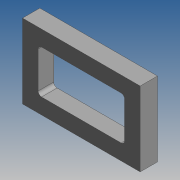
# Autodesk Inventor part: P031_MonoVitreBas
Saved by Autodesk Inventor 2021.3 (Build 253353000, 353)
## iProperties
Created: 2021-11-12
Part Number: P031_MonoVitreBas
Material: Générique
Document SubType Name: Modeling
Designer: gabri
Density: 1 g/cm^3
Appearance: Par défaut
Author: gabri
Autodesk Inventor part; units mm, degrees
ref_plane "YZ Plane" through (0, 0, 0) normal (1, 0, 0) x (0, 1, 0)
ref_plane "XZ Plane" through (0, 0, 0) normal (0, 1, 0) x (-1, 0, 0)
ref_plane "XY Plane" through (0, 0, 0) normal (0, 0, 1) x (1, 0, 0)
sketch "Sketch2" plane through (0, 0, 0) normal (0, 1, 0) x (-1, 0, 0)
  line L0 (-25, -12.5) -> (25, -12.5)
  line L1 (25, -12.5) -> (25, 12.5)
  line L2 (25, 12.5) -> (-25, 12.5)
  line L3 (-25, 12.5) -> (-25, -12.5)
  line L4 (-25, -12.5) -> (25, 12.5) construction
  line L5 (25, -12.5) -> (-25, 12.5) construction
  line L6 (-34, -21.5) -> (34, -21.5)
  line L7 (34, -21.5) -> (34, 21.5)
  line L8 (34, 21.5) -> (-34, 21.5)
  line L9 (-34, 21.5) -> (-34, -21.5)
  line L10 (-34, -21.5) -> (34, 21.5) construction
  line L11 (34, -21.5) -> (-34, 21.5) construction
  point P0 (0, 0)
  dimension "d0" = 50
  dimension "d1" = 25
  dimension "d4" = 9
  dimension "d5" = 9
  dimension "d53" = 68
  dimension "d54" = 43
  constraints: 24 end point, 4 midpoint, 4 parallel, 2 horizontal, 2 perpendicular
  measures "d0" distance of L1.end L2.end
  measures "d1" distance of L0.end L1.end
  measures "d4" distance between parallel lines of L8 L2
  measures "d5" distance between parallel lines of L1 L7
  measures "d53" distance of L6.start L6.end
  measures "d54" distance of L8.end L6.start
extrude "Extrusion1" add sketch "Sketch2" along normal blind 10
sketch "Sketch4" plane through (0, 10, 0) normal (0, 1, 0) x (1, 0, 0)
  line L0 (-34, 21.5) -> (-34, -21.5) construction
  line L1 (-34, -21.5) -> (34, -21.5) construction
  line L2 (34, -21.5) -> (34, 21.5) construction
  line L3 (34, 21.5) -> (-34, 21.5) construction
  line L4 (25, 12.5) -> (25, -12.5) construction
  line L5 (25, -12.5) -> (-25, -12.5) construction
  line L6 (-25, -12.5) -> (-25, 12.5) construction
  line L7 (-25, 12.5) -> (25, 12.5) construction
  line L8 (-25, 12.5) -> (25, 12.5)
  line L9 (25, 12.5) -> (25, -12.5)
  line L10 (25, -12.5) -> (-25, -12.5)
  line L11 (-25, -12.5) -> (-25, 12.5)
  line L12 (-25, 12.5) -> (25, -12.5) construction
  line L13 (25, 12.5) -> (-25, -12.5) construction
  line L14 (-29, 16.5) -> (29, 16.5)
  line L15 (29, 16.5) -> (29, -16.5)
  line L16 (29, -16.5) -> (-29, -16.5)
  line L17 (-29, -16.5) -> (-29, 16.5)
  line L18 (-29, 16.5) -> (29, -16.5) construction
  line L19 (29, 16.5) -> (-29, -16.5) construction
  point P0 (0, 0)
  dimension "d8" = 4
  dimension "d9" = 4
  constraints: 24 end point, 4 midpoint, 4 parallel, 2 horizontal, 2 perpendicular
  measures "d8" distance between parallel lines of L16 L10
  measures "d9" distance between parallel lines of L4 L15
extrude "Extrusion2" cut sketch "Sketch4" against normal blind 1
sketch "Sketch7" plane through (0, 9, 0) normal (0, 1, 0) x (1, 0, 0)
  line L0 (29, -16.5) -> (-29, -16.5) construction
  line L1 (29, 16.5) -> (29, -16.5) construction
  line L2 (-29, 16.5) -> (29, 16.5) construction
  line L3 (-29, -16.5) -> (-29, 16.5) construction
  line L4 (25, 12.5) -> (-25, 12.5) construction
  line L5 (25, -12.5) -> (25, 12.5) construction
  line L6 (-25, -12.5) -> (25, -12.5) construction
  line L7 (-25, 12.5) -> (-25, -12.5) construction
  line L8 (-26, 13.5) -> (26, 13.5)
  line L9 (26, 13.5) -> (26, -13.5)
  line L10 (26, -13.5) -> (-26, -13.5)
  line L11 (-26, -13.5) -> (-26, 13.5)
  line L12 (-26, 13.5) -> (26, -13.5) construction
  line L13 (26, 13.5) -> (-26, -13.5) construction
  line L14 (-29, 16.5) -> (29, 16.5)
  line L15 (29, 16.5) -> (29, -16.5)
  line L16 (29, -16.5) -> (-29, -16.5)
  line L17 (-29, -16.5) -> (-29, 16.5)
  line L18 (-29, 16.5) -> (29, -16.5) construction
  line L19 (29, 16.5) -> (-29, -16.5) construction
  point P0 (0, 0)
  dimension "d15" = 3
  dimension "d16" = 3
  constraints: 24 end point, 4 midpoint, 4 parallel, 2 horizontal, 2 perpendicular
  measures "d15" distance between parallel lines of L10 L0
  measures "d16" distance between parallel lines of L9 L15
extrude "Extrusion3" cut sketch "Sketch7" against normal blind 2.5
fillet "Fillet1" radius 2 8 edges at (26, 7.75, 13.5) (-26, 7.75, 13.5) (-26, 7.75, -13.5) (26, 7.75, -13.5) (25, 4.5, 12.5) (25, 4.5, -12.5) (-25, 4.5, -12.5) (-25, 4.5, 12.5)
fillet "Fillet2" radius 2 4 edges at (29, 8.25, 16.5) (29, 8.25, -16.5) (-29, 8.25, 16.5) (-29, 8.25, -16.5)
sketch "Sketch8" plane through (0, 10, 0) normal (0, 1, 0) x (1, 0, 0)
  line L0 (29, 14.5) -> (29, -14.5) construction
  arc A0 (27, -16.5) -> (29, -14.5) centre (27, -14.5) ccw construction
  line L1 (27, -16.5) -> (-27, -16.5) construction
  arc A1 (-29, -14.5) -> (-27, -16.5) centre (-27, -14.5) ccw construction
  line L2 (-29, -14.5) -> (-29, 14.5) construction
  arc A2 (-27, 16.5) -> (-29, 14.5) centre (-27, 14.5) ccw construction
  line L3 (-27, 16.5) -> (27, 16.5) construction
  arc A3 (29, 14.5) -> (27, 16.5) centre (27, 14.5) ccw construction
  line L4 (-34, 21.5) -> (-34, -21.5) construction
  line L5 (-34, -21.5) -> (34, -21.5) construction
  line L6 (34, -21.5) -> (34, 21.5) construction
  line L7 (34, 21.5) -> (-34, 21.5) construction
  line L8 (49, 0) -> (-49, 0) construction
  line L9 (0, 31.5) -> (0, -31.5) construction
  line L10 (-25, 10.5) -> (-25, -10.5) construction
  line L11 (23, 12.5) -> (-23, 12.5) construction
  line L12 (25, -10.5) -> (25, 10.5) construction
  line L13 (-23, -12.5) -> (23, -12.5) construction
  point P0 (0, 0)
  point P1 (31, -18.5)
  point P2 (31, 0)
  point P3 (31, 18.5)
  point P4 (0, 18.5)
  point P5 (-31, 18.5)
  point P6 (-31, 0)
  point P7 (-31, -18.5)
  point P8 (0, -18.5)
  dimension "d21" = 5
  dimension "d41" = 6
  dimension "d42" = 6
  dimension "d43" = 6
  dimension "d44" = 6
  dimension "d45" = 6
  dimension "d46" = 6
  dimension "d47" = 6
  dimension "d48" = 6
  dimension "d49" = 6
  dimension "d50" = 6
  dimension "d51" = 6
  dimension "d52" = 6
  constraints: 4 point on line
  measures "d21" distance between parallel lines of L7 L3
  measures "d41" distance from line of L10 point (-31, 18.5)
  measures "d42" distance from line of L11 point (-31, 18.5)
  measures "d43" distance from line of L11 point (0, 18.5)
  measures "d44" distance from line of L11 point (31, 18.5)
  measures "d45" distance from line of L12 point (31, 18.5)
  measures "d46" distance from line of L12 point (31, 0)
  measures "d47" distance from line of L13 point (31, -18.5)
  measures "d48" distance from line of L12 point (31, -18.5)
  measures "d49" distance from line of L13 point (0, -18.5)
  measures "d50" distance from line of L13 point (-31, -18.5)
  measures "d51" distance from line of L10 point (-31, -18.5)
  measures "d52" distance from line of L10 point (-31, 0)
hole "Hole1" at (31, 10, 18.5) at (31, 10, 0) at (31, 10, -18.5) at (0, 10, -18.5) at (-31, 10, -18.5) at (-31, 10, 0) at (-31, 10, 18.5) at (0, 10, 18.5) direction (0, -1, 0) diameter 2.459 depth 8.8 tip angle 118 thread size "M3x0.5" class "6H" standard "ISO Metric profile"
body "Solid1"
